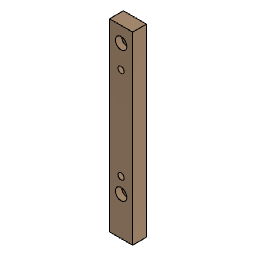
Standoff L (Autodesk Fusion 360 design; units mm, degrees)
Autodesk Fusion 360 part; units mm, degrees
sketch "Front" plane through (0, 0, 0) normal (0, 1, 0) x (1, 0, 0)
  line L0 (-15, -120) -> (15, -120)
  line L1 (15, -120) -> (15, 120)
  line L2 (15, 120) -> (-15, 120)
  line L3 (-15, 120) -> (-15, -120)
  line L4 (0, -120) -> (0, 120) construction
  circle A0 centre (0, -100) radius 4
  circle A1 centre (0, -70) radius 4
  circle A2 centre (0, 50) radius 4
  circle A3 centre (0, 70) radius 4
  circle A4 centre (0, -100) radius 7.5
  circle A5 centre (0, 70) radius 7.5
  dimension "d1" = 240
  dimension "d2" = 30
  dimension "d3" = 8
  dimension "d4" = 8
  dimension "d5" = 8
  dimension "d6" = 8
  dimension "d7" = 50
  dimension "d8" = 20
  dimension "d9" = 30
  dimension "d10" = 20
  dimension "d15" = 15
  dimension "d16" = 15
  constraint horizontal L0
  constraint vertical L1
  constraint horizontal L2
  constraint vertical L3
  constraint midpoint L0 L4.start
  constraint midpoint L2 L4.end
  constraint coincident L4 A0.centre
  constraint coincident L4 A1.centre
  constraint coincident L4 A2.centre
  constraint coincident L4 A3.centre
  constraint concentric A0 A4
  constraint concentric A3 A5
  measures "d1" distance of L0.start L2.end
  measures "d2" distance of L0.start L0.end
  measures "d3" diameter of A0
  measures "d4" diameter of A1
  measures "d5" diameter of A2
  measures "d6" diameter of A3
  measures "d7" distance of L2 A3.centre
  measures "d8" distance of A2.centre A3.centre
  measures "d9" distance of A0.centre A1.centre
  measures "d10" distance of L0 A0.centre
  measures "d15" diameter of A4
  measures "d16" diameter of A5
extrude "Extrude3" add sketch "Front" against normal blind 10 contours A4 | A5 makes body 1 at (7.4907, -6.6667, 100.3738) makes body 2 at (7.4907, -6.6667, -69.6262)
extrude "Extrude4" add sketch "Front" against normal blind 18 contours L0 L1 L2 L3 bodies 1 2
named bodies: "Standoff L"
